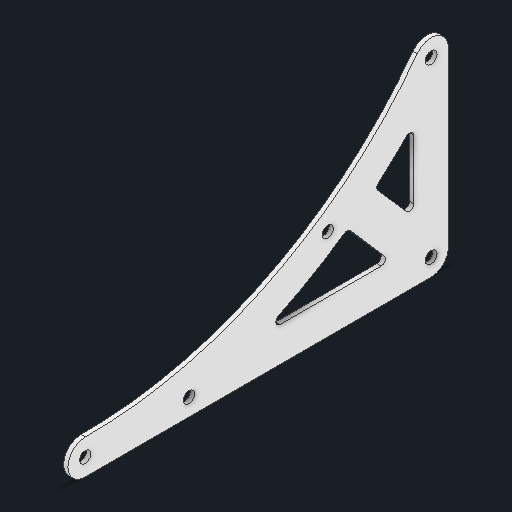
# Autodesk Inventor part: Scoop Gusset
Saved by Autodesk Inventor 2025.1 (Build 291241000, 241)
## iProperties
Created: 2024-10-25
Part Number: Scoop Gusset
Material: Acetal Resin, White
Document SubType Name: Modeling
Designer: avere
Density: 1.425 g/cm^3
Appearance: Smooth - White
Author: avere
Autodesk Inventor part; units mm, degrees
ref_plane "YZ Plane" through (0, 0, 0) normal (1, 0, 0) x (0, 1, 0)
ref_plane "XZ Plane" through (0, 0, 0) normal (0, 1, 0) x (-1, 0, 0)
ref_plane "XY Plane" through (0, 0, 0) normal (0, 0, 1) x (1, 0, 0)
sketch "main" plane through (0, 0, 0) normal (0, 0, 1) x (1, 0, 0)
  circle A0 centre (-72.2021, -58.7899) radius 2.1844
  circle A1 centre (-8.7021, -58.7899) radius 2.1844
  circle A2 centre (-72.2021, 68.2101) radius 2.0955
  arc A3 (-65.8522, 68.1715) -> (-78.5521, 68.2101) centre (-72.2021, 68.2101) ccw
  arc A4 (-78.5521, -58.7899) -> (-72.2021, -65.1399) centre (-72.2021, -58.7899) ccw
  arc A5 (-8.7021, -65.1399) -> (-4.923, -53.6869) centre (-8.7021, -58.7899) ccw
  line L0 (-8.7021, -65.1399) -> (-72.2021, -65.1399)
  line L1 (-78.5521, -58.7899) -> (-78.5521, 68.2101)
  arc A6 (-65.8522, 68.1715) -> (-4.923, -53.6869) centre (84.6432, 67.2577) ccw
  circle A7 centre (-45.1241, -20.8434) radius 2.0955
  circle A8 centre (-72.2021, 30.1101) radius 2.0955
  line L2 (-30.2668, -52.4399) -> (-52.0453, -52.4399)
  line L3 (-65.8521, -40.4491) -> (-65.8521, -3.317)
  line L4 (-65.8521, 68.1906) -> (-65.8521, 68.2101)
  arc A9 (-30.2668, -52.4399) -> (-29.1598, -49.7146) centre (-30.2668, -50.8524) ccw
  arc A10 (-62.8301, -2.6371) -> (-65.8521, -3.317) centre (-64.2646, -3.317) ccw
  line L5 (-63.2196, -41.6442) -> (-48.8544, -29.0826)
  line L6 (-53.0903, -49.6574) -> (-41.1491, -39.2154)
  arc A11 (-62.8301, -2.6371) -> (-48.6032, -26.9709) centre (84.6432, 67.2577) ccw
  arc A12 (-38.9023, -39.3732) -> (-29.1598, -49.7146) centre (84.6432, 67.2577) ccw
  arc A13 (-48.8544, -29.0826) -> (-48.6032, -26.9709) centre (-49.8994, -27.8875) ccw
  arc A14 (-65.8521, -40.4491) -> (-63.2196, -41.6442) centre (-64.2646, -40.4491) ccw
  arc A15 (-53.0903, -49.6574) -> (-52.0453, -52.4399) centre (-52.0453, -50.8524) ccw
  arc A16 (-38.9023, -39.3732) -> (-41.1491, -39.2154) centre (-40.1041, -40.4105) ccw
  point P0 (-46.4652, -14.2849)
  point P1 (-26.2898, -52.4399)
  point P2 (-65.8521, 4.1323)
  point P3 (-47.7717, -28.1358)
  point P4 (-39.9404, -38.1585)
  point P5 (-65.3871, -51.9749)
  dimension "d0" = 4.191
  dimension "d1" = 12.7
  dimension "d3" = 4.191
  dimension "d4" = 4.191
  dimension "d8" = 1.5875
  dimension "d9" = 12.7
  dimension "d10" = 6.35
  dimension "d11" = 1.5875
  measures "d0" diameter of A2
  measures "d1" diameter of A5
  measures "d3" diameter of A7
  measures "d4" diameter of A8
  measures "d8" radius of A9
  measures "d9" distance between parallel lines of L6 L5
  measures "d10" distance from line of point (-65.387, -51.975) L6
  measures "d11" radius of A13
sketch "Sketch1" plane through (0, 0, 0) normal (1, 0, 0) x (0, 1, 0)
  circle A0 centre (0, 0) radius 2.1844
  circle A1 centre (63.5, 0) radius 2.1844
  circle A2 centre (0, 127) radius 2.0955
  arc A3 (6.3499, 126.9614) -> (-6.35, 127) centre (0, 127) ccw
  arc A4 (-6.35, 0) -> (0, -6.35) centre (0, 0) ccw
  arc A5 (63.5, -6.35) -> (67.2791, 5.103) centre (63.5, 0) ccw
  line L0 (63.5, -6.35) -> (0, -6.35)
  line L1 (-6.35, 0) -> (-6.35, 127)
  arc A6 (6.3499, 126.9614) -> (67.2791, 5.103) centre (156.8453, 126.0476) ccw
  circle A7 centre (27.078, 37.9465) radius 2.0955
  circle A8 centre (0, 88.9) radius 2.0955
  line L2 (41.9353, 6.35) -> (20.1568, 6.35)
  line L3 (6.35, 18.3408) -> (6.35, 55.4729)
  line L4 (6.35, 126.9805) -> (6.35, 127)
  arc A9 (41.9353, 6.35) -> (43.0423, 9.0753) centre (41.9353, 7.9375) ccw
  arc A10 (9.372, 56.1528) -> (6.35, 55.4729) centre (7.9375, 55.4729) ccw
  line L5 (8.9825, 17.1457) -> (23.3477, 29.7074)
  line L6 (19.1118, 9.1325) -> (31.053, 19.5745)
  arc A11 (9.372, 56.1528) -> (23.5989, 31.819) centre (156.8453, 126.0476) ccw
  arc A12 (33.2998, 19.4167) -> (43.0423, 9.0753) centre (156.8453, 126.0476) ccw
  arc A13 (23.3477, 29.7074) -> (23.5989, 31.819) centre (22.3027, 30.9024) ccw
  arc A14 (6.35, 18.3408) -> (8.9825, 17.1457) centre (7.9375, 18.3408) ccw
  arc A15 (19.1118, 9.1325) -> (20.1568, 6.35) centre (20.1568, 7.9375) ccw
  arc A16 (33.2998, 19.4167) -> (31.053, 19.5745) centre (32.098, 18.3794) ccw
  constraints: 1 other
extrude "Extrusion1" add sketch "Sketch1" against normal blind 1.5875
body "Solid1"
